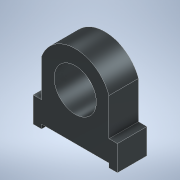
# Autodesk Inventor part: GuideSlider
Saved by Autodesk Inventor 2022.2 (Build 262287030, 287C)
## iProperties
Created: 2023-03-20
Part Number: GuideSlider
Material: Iron, Cast
Document SubType Name: Modeling
Designer: jak27277
Density: 7.15 g/cm^3
Appearance: Iron Gray
Author: jak27277
Autodesk Inventor part; units mm, degrees
ref_plane "YZ Plane" through (0, 0, 0) normal (1, 0, 0) x (0, 1, 0)
ref_plane "XZ Plane" through (0, 0, 0) normal (0, 1, 0) x (-1, 0, 0)
ref_plane "XY Plane" through (0, 0, 0) normal (0, 0, 1) x (1, 0, 0)
sketch "Sketch1" plane through (0, 0, 0) normal (0, 0, 1) x (1, 0, 0)
  line L0 (0, 0) -> (0, 152.8038)
  line L1 (-50.8, 94.6409) -> (-50.8, 38.3019)
  line L2 (-50.8, 38.3019) -> (-63.5, 38.3019)
  line L3 (-63.5, 38.3019) -> (-63.5, 0.2019)
  line L4 (-63.5, 0.2019) -> (-50.8, 0.2019)
  line L5 (-50.8, 0.2019) -> (-50.8, 6.5519)
  line L6 (-50.8, 6.5519) -> (0, 6.5519)
  line L7 (50.8, 94.6409) -> (50.8, 38.3019)
  line L8 (50.8, 38.3019) -> (63.5, 38.3019)
  line L9 (63.5, 38.3019) -> (63.5, 0.2019)
  line L10 (63.5, 0.2019) -> (50.8, 0.2019)
  line L11 (50.8, 0.2019) -> (50.8, 6.5519)
  line L12 (50.8, 6.5519) -> (0, 6.5519)
  circle A0 centre (0, 76.4019) radius 31.75
  arc A1 (50.8, 94.6409) -> (-50.8, 94.6409) centre (0, 76.4019) ccw
  dimension "d9" = 63.5
  dimension "d10" = 76.2
  dimension "d11" = 101.6
  dimension "d12" = 12.7
  dimension "d13" = 6.35
  dimension "d14" = 38.1
  dimension "d15" = 53.975
  constraints: 26 end point, 6 symmetric about line, 5 point on line, 4 perpendicular, 2 centre point, 2 midpoint, 2 point on circle, 2 vertical, 1 coincident, 1 horizontal
  measures "d9" diameter of A0
  measures "d10" distance from line of L4 A0.centre
  measures "d11" distance between parallel lines of L11 L5
  measures "d12" distance of L9.end L10.end
  measures "d13" distance between parallel lines of L10 L12
  measures "d14" distance of L8.end L9.end
  measures "d15" radius of A1
extrude "Extrusion1" add sketch "Sketch1" along normal blind 44.45 contours L6 L5 L4 L3 L2 L1 A1 L0 A0 | L0 A0 A1 L7 L8 L9 L10 L11 L12
body "Solid1"
